Autodesk Inventor part; units mm, degrees
(part 2 of 2)
  line L892 (5.6134, 13.843) -> (5.6134, 15.875) projected
  line L893 (5.6134, 15.875) -> (7.6454, 15.875) projected
  line L894 (7.6454, 15.875) -> (7.6454, 13.843) projected
  line L895 (7.6454, 13.843) -> (5.6134, 13.843) projected
  line L896 (5.6134, 11.303) -> (5.6134, 13.335) projected
  line L897 (5.6134, 13.335) -> (7.6454, 13.335) projected
  line L898 (7.6454, 13.335) -> (7.6454, 11.303) projected
  line L899 (7.6454, 11.303) -> (5.6134, 11.303) projected
  line L900 (5.6134, 8.763) -> (5.6134, 10.795) projected
  line L901 (5.6134, 10.795) -> (7.6454, 10.795) projected
  line L902 (7.6454, 10.795) -> (7.6454, 8.763) projected
  line L903 (7.6454, 8.763) -> (5.6134, 8.763) projected
  line L904 (3.0734, 31.623) -> (3.0734, 33.655) projected
  line L905 (3.0734, 33.655) -> (5.1054, 33.655) projected
  line L906 (5.1054, 33.655) -> (5.1054, 31.623) projected
  line L907 (5.1054, 31.623) -> (3.0734, 31.623) projected
  line L908 (3.0734, 29.083) -> (3.0734, 31.115) projected
  line L909 (3.0734, 31.115) -> (5.1054, 31.115) projected
  line L910 (5.1054, 31.115) -> (5.1054, 29.083) projected
  line L911 (5.1054, 29.083) -> (3.0734, 29.083) projected
  line L912 (3.0734, 26.543) -> (3.0734, 28.575) projected
  line L913 (3.0734, 28.575) -> (5.1054, 28.575) projected
  line L914 (5.1054, 28.575) -> (5.1054, 26.543) projected
  line L915 (5.1054, 26.543) -> (3.0734, 26.543) projected
  line L916 (3.0734, 24.003) -> (3.0734, 26.035) projected
  line L917 (3.0734, 26.035) -> (5.1054, 26.035) projected
  line L918 (5.1054, 26.035) -> (5.1054, 24.003) projected
  line L919 (5.1054, 24.003) -> (3.0734, 24.003) projected
  line L920 (3.0734, 21.463) -> (3.0734, 23.495) projected
  line L921 (3.0734, 23.495) -> (5.1054, 23.495) projected
  line L922 (5.1054, 23.495) -> (5.1054, 21.463) projected
  line L923 (5.1054, 21.463) -> (3.0734, 21.463) projected
  line L924 (3.0734, 18.923) -> (3.0734, 20.955) projected
  line L925 (3.0734, 20.955) -> (5.1054, 20.955) projected
  line L926 (5.1054, 20.955) -> (5.1054, 18.923) projected
  line L927 (5.1054, 18.923) -> (3.0734, 18.923) projected
  line L928 (3.0734, 16.383) -> (3.0734, 18.415) projected
  line L929 (3.0734, 18.415) -> (5.1054, 18.415) projected
  line L930 (5.1054, 18.415) -> (5.1054, 16.383) projected
  line L931 (5.1054, 16.383) -> (3.0734, 16.383) projected
  line L932 (3.0734, 13.843) -> (3.0734, 15.875) projected
  line L933 (3.0734, 15.875) -> (5.1054, 15.875) projected
  line L934 (5.1054, 15.875) -> (5.1054, 13.843) projected
  line L935 (5.1054, 13.843) -> (3.0734, 13.843) projected
  line L936 (3.0734, 11.303) -> (3.0734, 13.335) projected
  line L937 (3.0734, 13.335) -> (5.1054, 13.335) projected
  line L938 (5.1054, 13.335) -> (5.1054, 11.303) projected
  line L939 (5.1054, 11.303) -> (3.0734, 11.303) projected
  line L940 (3.0734, 8.763) -> (3.0734, 10.795) projected
  line L941 (3.0734, 10.795) -> (5.1054, 10.795) projected
  line L942 (5.1054, 10.795) -> (5.1054, 8.763) projected
  line L943 (5.1054, 8.763) -> (3.0734, 8.763) projected
  line L944 (0.5334, 31.623) -> (0.5334, 33.655) projected
  line L945 (0.5334, 33.655) -> (2.5654, 33.655) projected
  line L946 (2.5654, 33.655) -> (2.5654, 31.623) projected
  line L947 (2.5654, 31.623) -> (0.5334, 31.623) projected
  line L948 (0.5334, 29.083) -> (0.5334, 31.115) projected
  line L949 (0.5334, 31.115) -> (2.5654, 31.115) projected
  line L950 (2.5654, 31.115) -> (2.5654, 29.083) projected
  line L951 (2.5654, 29.083) -> (0.5334, 29.083) projected
  line L952 (0.5334, 26.543) -> (0.5334, 28.575) projected
  line L953 (0.5334, 28.575) -> (2.5654, 28.575) projected
  line L954 (2.5654, 28.575) -> (2.5654, 26.543) projected
  line L955 (2.5654, 26.543) -> (0.5334, 26.543) projected
  line L956 (0.5334, 24.003) -> (0.5334, 26.035) projected
  line L957 (0.5334, 26.035) -> (2.5654, 26.035) projected
  line L958 (2.5654, 26.035) -> (2.5654, 24.003) projected
  line L959 (2.5654, 24.003) -> (0.5334, 24.003) projected
  line L960 (0.5334, 21.463) -> (0.5334, 23.495) projected
  line L961 (0.5334, 23.495) -> (2.5654, 23.495) projected
  line L962 (2.5654, 23.495) -> (2.5654, 21.463) projected
  line L963 (2.5654, 21.463) -> (0.5334, 21.463) projected
  line L964 (0.5334, 18.923) -> (0.5334, 20.955) projected
  line L965 (0.5334, 20.955) -> (2.5654, 20.955) projected
  line L966 (2.5654, 20.955) -> (2.5654, 18.923) projected
  line L967 (2.5654, 18.923) -> (0.5334, 18.923) projected
  line L968 (0.5334, 16.383) -> (0.5334, 18.415) projected
  line L969 (0.5334, 18.415) -> (2.5654, 18.415) projected
  line L970 (2.5654, 18.415) -> (2.5654, 16.383) projected
  line L971 (2.5654, 16.383) -> (0.5334, 16.383) projected
  line L972 (0.5334, 13.843) -> (0.5334, 15.875) projected
  line L973 (0.5334, 15.875) -> (2.5654, 15.875) projected
  line L974 (2.5654, 15.875) -> (2.5654, 13.843) projected
  line L975 (2.5654, 13.843) -> (0.5334, 13.843) projected
  line L976 (0.5334, 11.303) -> (0.5334, 13.335) projected
  line L977 (0.5334, 13.335) -> (2.5654, 13.335) projected
  line L978 (2.5654, 13.335) -> (2.5654, 11.303) projected
  line L979 (2.5654, 11.303) -> (0.5334, 11.303) projected
  line L980 (0.5334, 8.763) -> (0.5334, 10.795) projected
  line L981 (0.5334, 10.795) -> (2.5654, 10.795) projected
  line L982 (2.5654, 10.795) -> (2.5654, 8.763) projected
  line L983 (2.5654, 8.763) -> (0.5334, 8.763) projected
  line L984 (0.5334, 6.223) -> (0.5334, 8.255) projected
  line L985 (0.5334, 8.255) -> (2.5654, 8.255) projected
  line L986 (2.5654, 8.255) -> (2.5654, 6.223) projected
  line L987 (2.5654, 6.223) -> (0.5334, 6.223) projected
  line L988 (0.5334, 3.683) -> (0.5334, 5.715) projected
  line L989 (0.5334, 5.715) -> (2.5654, 5.715) projected
  line L990 (2.5654, 5.715) -> (2.5654, 3.683) projected
  line L991 (2.5654, 3.683) -> (0.5334, 3.683) projected
  line L992 (0.5334, 1.143) -> (0.5334, 3.175) projected
  line L993 (0.5334, 3.175) -> (2.5654, 3.175) projected
  line L994 (2.5654, 3.175) -> (2.5654, 1.143) projected
  line L995 (2.5654, 1.143) -> (0.5334, 1.143) projected
  line L996 (0, 0) -> (51.7271, 0) projected
  line L997 (51.7271, 0) -> (51.7271, 34.1376) projected
  line L998 (51.7271, 34.1376) -> (0, 34.1376) projected
  line L999 (0, 34.1376) -> (0, 0) projected
  circle A3 centre (1.5494, 4.699) radius 0.508 projected
  circle A4 centre (1.5494, 7.239) radius 0.508 projected
  circle A5 centre (1.5494, 9.779) radius 0.508 projected
  circle A6 centre (1.5494, 12.319) radius 0.508 projected
  circle A7 centre (1.5494, 14.859) radius 0.508 projected
  circle A8 centre (1.5494, 17.399) radius 0.508 projected
  circle A9 centre (1.5494, 19.939) radius 0.508 projected
  circle A10 centre (1.5494, 22.479) radius 0.508 projected
  circle A11 centre (1.5494, 25.019) radius 0.508 projected
  circle A12 centre (1.5494, 27.559) radius 0.508 projected
  circle A13 centre (1.5494, 30.099) radius 0.508 projected
  circle A14 centre (1.5494, 32.639) radius 0.508 projected
  circle A15 centre (4.0894, 32.639) radius 0.508 projected
  circle A16 centre (6.6294, 32.639) radius 0.508 projected
  circle A17 centre (9.1694, 32.639) radius 0.508 projected
  circle A18 centre (11.7094, 32.639) radius 0.508 projected
  circle A19 centre (14.2494, 32.639) radius 0.508 projected
  circle A20 centre (16.7894, 32.639) radius 0.508 projected
  circle A21 centre (19.3294, 32.639) radius 0.508 projected
  circle A22 centre (21.8694, 32.639) radius 0.508 projected
  circle A23 centre (24.4094, 32.639) radius 0.508 projected
  line L1000 (27.9654, 31.623) -> (27.9654, 33.655) projected
  circle A24 centre (26.9494, 32.639) radius 0.508 projected
  line L1001 (30.5054, 31.623) -> (30.5054, 33.655) projected
  circle A25 centre (29.4894, 32.639) radius 0.508 projected
  circle A26 centre (32.0294, 32.639) radius 0.508 projected
  circle A27 centre (34.5694, 32.639) radius 0.508 projected
  circle A28 centre (37.1094, 32.639) radius 0.508 projected
  circle A29 centre (39.6494, 32.639) radius 0.508 projected
  circle A30 centre (42.1894, 32.639) radius 0.508 projected
  circle A31 centre (44.7294, 32.639) radius 0.508 projected
  circle A32 centre (47.2694, 32.639) radius 0.508 projected
  circle A33 centre (49.8094, 32.639) radius 0.508 projected
  circle A34 centre (49.8094, 30.099) radius 0.508 projected
  circle A35 centre (49.8094, 27.559) radius 0.508 projected
  line L1002 (50.8254, 26.035) -> (48.7934, 26.035) projected
  circle A36 centre (49.8094, 25.019) radius 0.508 projected
  circle A37 centre (49.8094, 22.479) radius 0.508 projected
  circle A38 centre (49.8094, 19.939) radius 0.508 projected
  circle A39 centre (49.8094, 17.399) radius 0.508 projected
  circle A40 centre (49.8094, 14.859) radius 0.508 projected
  circle A41 centre (49.8094, 12.319) radius 0.508 projected
  circle A42 centre (49.8094, 9.779) radius 0.508 projected
  circle A43 centre (49.8094, 7.239) radius 0.508 projected
  circle A44 centre (49.8094, 4.699) radius 0.508 projected
  circle A45 centre (49.8094, 2.159) radius 0.508 projected
  line L1003 (48.2854, 3.175) -> (46.2534, 3.175) projected
  circle A46 centre (47.2694, 2.159) radius 0.508 projected
  circle A47 centre (44.7294, 2.159) radius 0.508 projected
  circle A48 centre (42.1894, 2.159) radius 0.508 projected
  circle A49 centre (39.6494, 2.159) radius 0.508 projected
  circle A50 centre (37.1094, 2.159) radius 0.508 projected
  circle A51 centre (34.5694, 2.159) radius 0.508 projected
  circle A52 centre (32.0294, 2.159) radius 0.508 projected
  circle A53 centre (29.4894, 2.159) radius 0.508 projected
  circle A54 centre (26.9494, 2.159) radius 0.508 projected
  circle A55 centre (24.4094, 2.159) radius 0.508 projected
  circle A56 centre (21.8694, 2.159) radius 0.508 projected
  circle A57 centre (19.3294, 2.159) radius 0.508 projected
  circle A58 centre (16.7894, 2.159) radius 0.508 projected
  circle A59 centre (14.2494, 2.159) radius 0.508 projected
  line L1004 (13.2334, 1.143) -> (50.8254, 1.143)
  line L1005 (50.8254, 1.143) -> (50.8254, 3.175)
  line L1006 (50.8254, 3.175) -> (13.2334, 3.175)
  line L1007 (13.2334, 3.175) -> (13.2334, 1.143)
  line L1008 (48.7934, 31.115) -> (50.8254, 31.115)
  line L1009 (50.8254, 31.115) -> (50.8254, 1.143)
  line L1010 (50.8254, 1.143) -> (48.7934, 1.143)
  line L1011 (48.7934, 1.143) -> (48.7934, 31.115)
  line L1012 (2.5654, 1.143) -> (0.5334, 1.143) projected
  line L1013 (2.5654, 1.143) -> (0.5334, 1.143)
  line L1014 (0.5334, 1.143) -> (0.5334, 33.655)
  line L1015 (0.5334, 33.655) -> (2.5654, 33.655)
  line L1016 (2.5654, 33.655) -> (2.5654, 1.143)
  line L1017 (0.5334, 33.655) -> (50.8254, 33.655)
  line L1018 (50.8254, 33.655) -> (50.8254, 31.623)
  line L1019 (50.8254, 31.623) -> (0.5334, 31.623)
  line L1020 (0.5334, 31.623) -> (0.5334, 33.655)
  constraints: 32 end point, 8 parallel, 4 horizontal, 4 perpendicular
extrude "Extrusion9" add sketch "Sketch9" along normal blind 0.0254 contours L1014 L991 L1016 L2 | L1014 L987 L1016 L989 | L1014 L983 L1016 L985 | L1014 L979 L1016 L981 | L1014 L975 L1016 L977 | L1014 L971 L1016 L973 | L1014 L967 L1016 L969 | L1014 L963 L1016 L965 | L1014 L959 L1016 L961 | L1014 L955 L1016 L957 | L1014 L951 L1016 L953 | L1014 L947 L1016 L949 | L946 L1017 L904 L1019 | L906 L1017 L864 L1019 | L866 L1017 L816 L1019 | L818 L1017 L768 L1019 | L770 L1017 L716 L1019 | L718 L1017 L664 L1019 | L666 L1017 L612 L1019 | L614 L1017 L560 L1019 | L562 L1017 L508 L1019 | L510 L1017 L456 L1019 | L458 L1017 L404 L1019 | L406 L1017 L352 L1019 | L354 L1017 L300 L1019 | L302 L1017 L248 L1019 | L250 L1017 L196 L1019 | L198 L1017 L144 L1019 | L146 L1017 L100 L1019 | L102 L1017 L56 L1019 | L58 L1017 L4 L1019 | L11 L1009 L13 L1011 | L15 L1009 L17 L1011 | L19 L1009 L21 L1011 | L23 L1009 L25 L1011 | L27 L1009 L29 L1011 | L31 L1009 L33 L1011 | L35 L1009 L37 L1011 | L39 L1009 L41 L1011 | L43 L1009 L45 L1011 | L47 L1009 L49 L1011 | L51 L1009 L53 L1011 | L52 L1004 L98 L1006 | L96 L1004 L142 L1006 | L140 L1004 L194 L1006 | L192 L1004 L246 L1006 | L244 L1004 L298 L1006 | L296 L1004 L350 L1006 | L348 L1004 L402 L1006 | L400 L1004 L454 L1006 | L452 L1004 L506 L1006 | L504 L1004 L558 L1006 | L556 L1004 L610 L1006 | L608 L1004 L662 L1006 | L660 L1004 L714 L1006 | L712 L1004 L766 L1006
equation "\"d3\" = d2"
body "Solid1"
